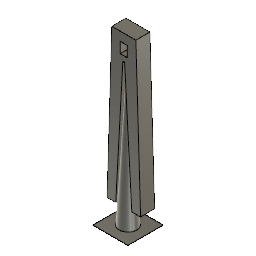
bear_short_layer (Autodesk Fusion 360 design; units mm, degrees)
Autodesk Fusion 360 part; units mm, degrees
sketch "Sketch1" plane through (0, 0, 0) normal (0, 1, 0) x (1, 0, 0) in component "spike"
  line L0 (0, 0) -> (5, 0)
  line L1 (5, 0) -> (0.45, -80)
  line L2 (0, -80) -> (0, 0)
  line L3 (0.45, -80) -> (0, -80)
  dimension "d1" = 5
  dimension "d8" = 0.45
  dimension "d9" = 80
  constraint coincident L0.start L2.end
  constraint horizontal L0
  constraint perpendicular L0 L2
  constraint perpendicular L2 L3
  measures "d1" distance of L0.start L0.end
  measures "d8" distance of L1.end L2.start
  measures "d9" distance of L0 L3
revolve "Revolve1" add sketch "Sketch1" angle 360 about axis through (0, 0, 80) along (0, 0, -1) makes body 1 in component "spike"
sketch "Sketch2" plane through (0, 0, 0) normal (0, 0, -1) x (1, 0, 0) in component "spike"
  circle A0 centre (0, 0) radius 5
  line L0 (10, 10) -> (-10, 10)
  line L1 (-10, 10) -> (-10, -10)
  line L2 (-10, -10) -> (10, -10)
  line L3 (10, -10) -> (10, 10)
  line L4 (10, 10) -> (-10, -10) construction
  line L5 (-10, 10) -> (10, -10) construction
  dimension "d4" = 20
  dimension "d5" = 20
  constraint perpendicular L0 L1
  constraint parallel L0 L2
  constraint parallel L1 L3
  constraint horizontal L0
  constraint coincident L4 A0.centre
  constraint coincident L5 A0.centre
  constraint coincident A0.centre origin
  measures "d4" distance of L0.end L1.end
  measures "d5" distance of L1.end L2.end
extrude "Extrude1" add sketch "Sketch2" against normal blind 0.2 contours A0 | L0 L1 L2 L3 bodies 1 in component "spike"
sketch "Sketch1 (2)" plane through (0, 0, 0) normal (0, 1, 0) x (1, 0, 0) in component "spike_measure_tool"
  line L0 (5, 0) -> (0.45, -80)
  line L1 (0, 0) -> (5, 0)
  line L2 (0, -80) -> (0, 0)
  line L3 (0.45, -80) -> (0, -80)
  line L4 (-0.45, -80) -> (0, -80)
  line L5 (6.8437, -95) -> (0, -95)
  line L6 (2, -90) -> (-2, -90)
  line L7 (-2, -90) -> (-2, -84)
  line L8 (-2, -84) -> (2, -84)
  line L9 (2, -84) -> (2, -90)
  line L10 (0, -80) -> (0, -84) construction
  line L11 (9.5, -10) -> (6.8437, -95)
  line L12 (2, -90) -> (7, -90) construction
  line L13 (-2, -90) -> (-7, -90) construction
  line L14 (9.5, -10) -> (0, -10)
  line L15 (0, -90) -> (0, -95) construction
  line L16 (4.5314, -10) -> (0.4933, -81)
  line L17 (0.4933, -81) -> (0, -81)
  line L18 (-4.5314, -10) -> (-0.4933, -81)
  line L19 (-9.5, -10) -> (-6.8438, -95)
  line L20 (-9.5, -10) -> (0, -10)
  line L21 (-6.8438, -95) -> (0, -95)
  line L22 (-0.4933, -81) -> (0, -81)
  point P0 (4.4312, -10)
  dimension "d13" = 4
  dimension "d14" = 6
  dimension "d16" = 5
  dimension "d17" = 5
  dimension "d53" = 10
  dimension "d54" = 90
  dimension "d55" = 9.5
  dimension "d56" = 0.1
  dimension "d57" = 1
  constraint symmetric L2 L0.end L4.start
  constraint symmetric L2 L3.end L4.end
  constraint horizontal L6
  constraint vertical L7
  constraint horizontal L8
  constraint vertical L9
  constraint midpoint L8 L10.end
  constraint vertical L10
  constraint coincident L11 L12.end
  constraint perpendicular L9 L12
  constraint perpendicular L7 L13
  constraint equal L12 L13
  constraint horizontal L14
  constraint coincident L14 P0
  constraint coincident L0 P0
  constraint coincident L2 L14.end
  constraint midpoint L6 L15.start
  constraint perpendicular L5 L15
  constraint coincident L14 L16.start
  constraint coincident L10 L17.end
  constraint perpendicular L10 L17
  constraint parallel L0 L16
  constraint symmetric L2 L11.start L19.start
  constraint symmetric L2 L5.start L19.end
  constraint symmetric L2 L5.end L15.end
  constraint symmetric L2 L14.end L20.end
  constraint symmetric L2 L16.start L18.start
  constraint symmetric L2 L16.end L18.end
  constraint symmetric L10 L16.end L18.end
  constraint symmetric L10 L17.end L22.end
  measures "d13" distance of L6.start L6.end
  measures "d14" distance of L6.end L7.end
  measures "d16" distance of L5 L6
  measures "d17" distance of L6.start L12.end
  measures "d53" distance of L1 L14
  measures "d54" distance of L1 L6
  measures "d55" horizontal distance of L1.start L11.start
  measures "d56" distance of L0 L16
  measures "d57" distance of L3 L17
extrude "Extrude1'" add sketch "Sketch1 (2)" along normal blind 8 separate body contours L0 L2 L3 L14 L16 L17 L18 L20 L22 | L0 L2 L3 L14 | L5 L11 L14 L16 L17 L18 L19 L20 L21 L22 makes body 2 in component "spike_measure_tool"
extrude "Extrude2" add sketch "Sketch1 (2)" along normal blind 1 contours L0 L2 L3 L14 L16 L17 L18 L20 L22 | L0 L2 L3 L14 bodies 2 in component "spike_measure_tool"
ref_plane "WorkPlane1" through (0, 2.4, 52.5) normal (0, 1, 0) x (0, 0, 1) in component "spike_measure_tool"
sketch "Sketch3" plane through (0, 2.4, 52.5) normal (0, 1, 0) x (1, 0, 0) in component "spike_measure_tool"
  line L0 (-4.5314, 42.5) -> (-0.4933, -28.5)
  line L1 (4.5314, 42.5) -> (0.4933, -28.5)
  line L2 (0.4933, -28.5) -> (0, -28.5)
  line L3 (-0.4933, -28.5) -> (0, -28.5)
  line L4 (9.5, 42.5) -> (-9.5, 42.5)
  line L5 (0, -28.5) -> (0, 42.5)
  constraint coincident L2.end L3.end
  constraint midpoint L4 L5.end
extrude "Extrude3" cut sketch "Sketch3" against normal blind 13 bodies 2 in component "spike_measure_tool"
revolve "Revolve2" cut sketch "Sketch3" angle 360 about axis through (0, 2.4, 81) along (0, 0, -1) contours L0 L3 L4 L5 bodies 2 in component "spike_measure_tool"
component "spike" placed x (1, 0, 0) y (0, 1, 0) z (0, 0, 1) at (0, 2.4, 0)
component "spike_measure_tool" placed x (1, 0, 0) y (0, 1, 0) z (0, 0, 1) at (0, 0, 0)
equation "d1 = spike_base_dia / 2"
equation "d9 = spike_height"
equation "spike_base_dia = 10 mm"
equation "spike_height = 80 mm"
equation "d47 = -0.6 mm - spike_base_dia / 2"
